Autodesk Fusion 360 part; units mm, degrees
(part 3 of 5)
sketch "Boceto1" plane through (0, 0, 0) normal (0, 1, 0) x (1, 0, 0)
  circle A0 centre (0, -615) radius 600 construction
  line L0 (0, 0) -> (-145, 0) construction
  circle A1 centre (-180, 0) radius 35 construction
  arc A2 (-148.5274, -15.3125) -> (-149.6891, 17.5) centre (-180, 0) ccw
  line L1 (-180, 0) -> (-153.1905, -22.5) construction
  line L2 (-180, 0) -> (-167.0096, 32.5) construction
  line L3 (-126.7013, 30.7139) -> (-107.5227, 7.8577)
  line L4 (-128.2, 32.5) -> (-139.7703, 32.5) construction
  line L5 (-138, 31.5) -> (-138, 5)
  line L6 (-138, 5) -> (-133.2, 5)
  line L7 (-133.2, 5) -> (-133.2, 31.25)
  line L8 (-141.0289, 32.5) -> (-139, 32.5)
  line L9 (-131.95, 32.5) -> (-130.5315, 32.5)
  line L10 (-145, 0) -> (-145, 32.5) construction
  line L11 (-35, -5) -> (-109.7758, -5)
  line L12 (-115.9041, -7.8577) -> (-125.7926, -19.6423)
  line L13 (-131.9209, -22.5) -> (-144.0313, -22.5)
  line L14 (-128.2, 19.2264) -> (-128.2, 7)
  line L15 (-126.2, 5) -> (-115.9408, 5)
  line L16 (-114.4087, 8.2856) -> (-124.6679, 20.512)
  arc A3 (-148.5274, -15.3125) -> (-144.0313, -22.5) centre (-144.0313, -17.5) ccw
  arc A4 (-141.0289, 32.5) -> (-149.6891, 17.5) centre (-141.0289, 22.5) ccw
  arc A5 (-128.2, 7) -> (-126.2, 5) centre (-126.2, 7) ccw
  arc A6 (-115.9408, 5) -> (-114.4087, 8.2856) centre (-115.9408, 7) ccw
  arc A7 (-124.6679, 20.512) -> (-128.2, 19.2264) centre (-126.2, 19.2264) ccw
  line L17 (-131.7, -16.1564) -> (-131.7, -1)
  line L18 (-129.934, -16.7992) -> (-117.2162, -1.6428)
  line L19 (-130.7, 0) -> (-117.9823, 0)
  arc A8 (-131.7, -16.1564) -> (-129.934, -16.7992) centre (-130.7, -16.1564) ccw
  arc A9 (-117.2162, -1.6428) -> (-117.9823, 0) centre (-117.9823, -1) ccw
  arc A10 (-130.7, 0) -> (-131.7, -1) centre (-130.7, -1) ccw
  line L20 (-138, 31.5) -> (-139, 32.5)
  line L21 (-133.2, 31.25) -> (-131.95, 32.5)
  arc A11 (-131.9209, -22.5) -> (-125.7926, -19.6423) centre (-131.9209, -14.5) ccw
  arc A12 (-109.7758, -5) -> (-115.9041, -7.8577) centre (-109.7758, -13) ccw
  arc A13 (-107.5227, 7.8577) -> (-101.3943, 5) centre (-101.3943, 13) ccw
  arc A14 (-126.7013, 30.7139) -> (-130.5315, 32.5) centre (-130.5315, 27.5) ccw
  line L22 (0, 105) -> (-30, 105)
  line L23 (-22, -14.9217) -> (-22, 0)
  line L24 (-22, 0) -> (-17.2, 0)
  line L25 (-17.2, 0) -> (-17.2, -14.7323)
  arc A15 (0, -15) -> (-16.6861, -15.2321) centre (0, -615) ccw
  arc A16 (-22.4813, -15.4213) -> (-26.8657, -15.6018) centre (0, -615) ccw
  line L26 (-30, -10) -> (-30, -12.6048)
  arc A17 (-30, -10) -> (-35, -5) centre (-35, -10) ccw
  arc A18 (-30, -12.6048) -> (-26.8657, -15.6018) centre (-27, -12.6048) ccw
  line L27 (0, 105) -> (0, -15)
  circle A19 centre (-143.9289, 24) radius 2.5
  circle A20 centre (-140.0313, -14.5) radius 4
  circle A21 centre (-138.0313, -4.5) radius 2.5
  line L28 (0, -1.75) -> (0, -22.5)
  arc A22 (149.6891, 17.5) -> (141.0289, 32.5) centre (141.0289, 22.5) ccw
  arc A23 (149.6891, 17.5) -> (148.5274, -15.3125) centre (180, 0) ccw
  circle A24 centre (143.9289, 24) radius 2.5
  line L29 (141.0289, 32.5) -> (139, 32.5)
  line L30 (138, 31.5) -> (139, 32.5)
  line L31 (138, 31.5) -> (138, 5)
  line L32 (133.2, 5) -> (133.2, 31.25)
  line L33 (138, 5) -> (133.2, 5)
  line L34 (133.2, 31.25) -> (131.95, 32.5)
  arc A25 (130.5315, 32.5) -> (126.7013, 30.7139) centre (130.5315, 27.5) ccw
  line L35 (131.95, 32.5) -> (130.5315, 32.5)
  arc A26 (128.2, 19.2264) -> (124.6679, 20.512) centre (126.2, 19.2264) ccw
  line L36 (128.2, 19.2264) -> (128.2, 7)
  line L37 (114.4087, 8.2856) -> (124.6679, 20.512)
  line L38 (126.7013, 30.7139) -> (107.5227, 7.8577)
  arc A27 (114.4087, 8.2856) -> (115.9408, 5) centre (115.9408, 7) ccw
  line L39 (126.2, 5) -> (115.9408, 5)
  arc A28 (126.2, 5) -> (128.2, 7) centre (126.2, 7) ccw
  circle A29 centre (138.0313, -4.5) radius 2.5
  arc A30 (131.7, -1) -> (130.7, 0) centre (130.7, -1) ccw
  line L40 (131.7, -16.1564) -> (131.7, -1)
  arc A31 (117.9823, 0) -> (117.2162, -1.6428) centre (117.9823, -1) ccw
  line L41 (130.7, 0) -> (117.9823, 0)
  line L42 (129.934, -16.7992) -> (117.2162, -1.6428)
  arc A32 (129.934, -16.7992) -> (131.7, -16.1564) centre (130.7, -16.1564) ccw
  circle A33 centre (140.0313, -14.5) radius 4
  arc A34 (144.0313, -22.5) -> (148.5274, -15.3125) centre (144.0313, -17.5) ccw
  line L43 (131.9209, -22.5) -> (144.0313, -22.5)
  arc A35 (125.7926, -19.6423) -> (131.9209, -22.5) centre (131.9209, -14.5) ccw
  line L44 (115.9041, -7.8577) -> (125.7926, -19.6423)
  arc A36 (115.9041, -7.8577) -> (109.7758, -5) centre (109.7758, -13) ccw
  line L45 (35, -5) -> (109.7758, -5)
  arc A37 (101.3943, 5) -> (107.5227, 7.8577) centre (101.3943, 13) ccw
  arc A38 (35, -5) -> (30, -10) centre (35, -10) ccw
  arc A39 (26.8657, -15.6018) -> (30, -12.6048) centre (27, -12.6048) ccw
  line L46 (30, -10) -> (30, -12.6048)
  arc A40 (26.8657, -15.6018) -> (22.4813, -15.4213) centre (0, -615) ccw
  line L47 (22, -14.9217) -> (22, 0)
  arc A41 (16.6861, -15.2321) -> (0, -15) centre (0, -615) ccw
  line L48 (17.2, 0) -> (17.2, -14.7323)
  line L49 (0, 0) -> (145, 0) construction
  line L50 (0, 105) -> (30, 105)
  line L51 (17.2, 0) -> (22, 0)
  arc A42 (-22.4813, -15.4213) -> (-22, -14.9217) centre (-22.5, -14.9217) ccw
  arc A43 (-17.2, -14.7323) -> (-16.6861, -15.2321) centre (-16.7, -14.7323) ccw
  arc A44 (16.6861, -15.2321) -> (17.2, -14.7323) centre (16.7, -14.7323) ccw
  arc A45 (22, -14.9217) -> (22.4813, -15.4213) centre (22.5, -14.9217) ccw
  line L52 (-22, -8) -> (-17.2, -8)
  line L53 (17.2, -8) -> (22, -8)
  line L54 (-52.8349, 8.75) -> (-34.6651, 40.2211)
  line L55 (-56.4434, 12.5) -> (-32.0096, 54.8205)
  line L56 (-101.3943, 5) -> (-69.4338, 5)
  line L57 (-50.6699, 5) -> (-32.5, 5)
  line L58 (-30, 105) -> (-30, 62.3205)
  line L59 (-30, 38.9711) -> (-30, 7.5)
  arc A46 (-69.4338, 5) -> (-56.4434, 12.5) centre (-69.4338, 20) ccw
  arc A47 (-32.0096, 54.8205) -> (-30, 62.3205) centre (-45, 62.3205) ccw
  arc A48 (-30, 38.9711) -> (-34.6651, 40.2211) centre (-32.5, 38.9711) ccw
  arc A49 (-32.5, 5) -> (-30, 7.5) centre (-32.5, 7.5) ccw
  arc A50 (-52.8349, 8.75) -> (-50.6699, 5) centre (-50.6699, 7.5) ccw
  line L60 (30, 105) -> (30, 62.3205)
  arc A51 (30, 62.3205) -> (32.0096, 54.8205) centre (45, 62.3205) ccw
  line L61 (56.4434, 12.5) -> (32.0096, 54.8205)
  arc A52 (34.6651, 40.2211) -> (30, 38.9711) centre (32.5, 38.9711) ccw
  line L62 (30, 38.9711) -> (30, 7.5)
  arc A53 (30, 7.5) -> (32.5, 5) centre (32.5, 7.5) ccw
  line L63 (50.6699, 5) -> (32.5, 5)
  arc A54 (50.6699, 5) -> (52.8349, 8.75) centre (50.6699, 7.5) ccw
  line L64 (52.8349, 8.75) -> (34.6651, 40.2211)
  arc A55 (56.4434, 12.5) -> (69.4338, 5) centre (69.4338, 20) ccw
  line L65 (101.3943, 5) -> (69.4338, 5)
  line L66 (50.6699, 5) -> (32.5, 5)
  point P0 (-167.0096, 32.5)
  point P1 (-138, 32.5)
  point P2 (-133.2, 32.5)
  point P3 (-128.1905, -22.5)
  point P4 (-30, 5)
  point P5 (-55, 5)
  dimension "d1" = 1200
  dimension "d13" = 70
  dimension "d21" = 50
  dimension "d23" = 5
  dimension "d25" = 4.8
  dimension "d26" = 7
  dimension "d27" = 5
  dimension "d28" = 5
  dimension "d29" = 25
  dimension "d30" = 50
  dimension "d31" = 55
  dimension "d32" = 32.5
  dimension "d33" = 5
  dimension "d34" = 5
  dimension "d35" = 10
  dimension "d36" = 2
  dimension "d37" = 32.5
  dimension "d39" = 5
  dimension "d40" = 1
  dimension "d44" = 1
  dimension "d45" = 1
  dimension "d46" = 1.25
  dimension "d47" = 1.25
  dimension "d48" = 8
  dimension "d49" = 5
  dimension "d50" = 5
  dimension "d52" = 30
  dimension "d53" = 600
  dimension "d54" = 4.8
  dimension "d55" = 8
  dimension "d57" = 5
  dimension "d58" = 3
  dimension "d59" = 120
  dimension "d72" = 1.5
  dimension "d73" = 5
  dimension "d74" = 2.9
  dimension "d75" = 1.5
  dimension "d76" = 8
  dimension "d78" = 4
  dimension "d79" = 3
  dimension "d80" = 5
  dimension "d81" = 10
  dimension "d82" = 2
  dimension "d83" = 615
  dimension "d84" = 0.5
  dimension "d85" = 7
  dimension "d86" = 7
  dimension "d87" = 60
  dimension "d88" = 25
  dimension "d89" = 5
  dimension "d90" = 15
  dimension "d91" = 2.5
  dimension "d166" = 180
  constraint coincident L0 A1.centre
  constraint coincident L0.end A1
  constraint coincident L49.start L0
  constraint coincident L0.start L49.start
  constraint coincident A1 P0
  constraint coincident A1.centre A2.centre
  constraint parallel L0 L8
  constraint horizontal L4
  constraint perpendicular L5 L8
  constraint perpendicular L5 L6
  constraint perpendicular L7 L9
  constraint collinear L8 L9
  constraint coincident L8 L10.end
  constraint tangent A2 L10
  constraint parallel L0 L11
  constraint horizontal L13
  constraint perpendicular L4 L14
  constraint perpendicular L14 L15
  constraint parallel L3 L16
  constraint coincident L6.end L15
  constraint coincident L4.start L14
  constraint coincident L1.end L13
  constraint coincident L1.end A2
  constraint tangent L13 A3
  constraint tangent A2 A3
  constraint coincident P0 L2.end
  constraint tangent L8 A4
  constraint tangent A2 A4
  constraint tangent L14 A5
  constraint tangent L15 A5
  constraint tangent L15 A6
  constraint tangent L16 A6
  constraint equal A5 A6
  constraint tangent L14 A7
  constraint tangent L16 A7
  constraint equal A5 A7
  constraint perpendicular L0 L17
  constraint parallel L12 L18
  constraint tangent L17 A8
  constraint tangent L18 A8
  constraint tangent L18 A9
  constraint tangent L19 A9
  constraint equal A8 A9
  constraint tangent L17 A10
  constraint tangent L19 A10
  constraint equal A8 A10
  constraint coincident L0 L19.start
  constraint horizontal L19
  constraint coincident P1 L5
  constraint coincident P1 L8
  constraint coincident P2 L7
  constraint coincident P2 L9
  constraint coincident P3 L12
  constraint coincident P3 L13
  constraint tangent L12 A11
  constraint tangent L13 A11
  constraint tangent L11 A12
  constraint tangent L12 A12
  constraint equal A11 A12
  constraint tangent L3 A13
  constraint tangent A13 L56
  constraint equal A11 A13
  constraint coincident L4.start L9
  constraint coincident L4.start L3
  constraint tangent L9 A14
  constraint tangent L3 A14
  constraint horizontal L22
  constraint vertical L58
  constraint coincident A0 A15.start
  constraint vertical L23
  constraint perpendicular L23 L24
  constraint vertical L25
  constraint concentric A15 A16
  constraint coincident L0.start L24
  constraint collinear L26 L59
  constraint tangent L11 A17
  constraint tangent L26 A17
  constraint tangent A16 A18
  constraint tangent L26 A18
  constraint coincident A15 L27.end
  constraint coincident L0.start L27
  constraint coincident A0.centre L28
  constraint vertical L27
  constraint symmetric L0.start L27 L49.start
  constraint symmetric L0.end L27 L49.end
  constraint symmetric A2 L27 A23
  constraint symmetric L5.end L27 L31.end
  constraint symmetric L6.end L27 L32.start
  constraint symmetric L13.end L27 A34.start
  constraint symmetric A2.start L27 A23.end
  constraint symmetric A3 L27 A34
  constraint symmetric L8.start L27 A22.end
  constraint symmetric A2.end L27 A22.start
  constraint symmetric A4 L27 A22
  constraint symmetric L14.end L27 L36.end
  constraint symmetric L15.start L27 L39.start
  constraint symmetric A5 L27 A28
  constraint symmetric L15.end L27 A27.end
  constraint symmetric L16.start L27 L37.start
  constraint symmetric A6 L27 A27
  constraint symmetric L14.start L27 A26.start
  constraint symmetric L16.end L27 A26.end
  constraint symmetric A7 L27 A26
  constraint symmetric L17.start L27 L40.start
  constraint symmetric L18.start L27 L42.start
  constraint symmetric A8 L27 A32
  constraint symmetric L18.end L27 A31.end
  constraint symmetric L19.end L27 A31.start
  constraint symmetric A9 L27 A31
  constraint symmetric L17.end L27 A30.start
  constraint symmetric L19.start L27 A30.end
  constraint symmetric A10 L27 A30
  constraint symmetric L5.start L27 L30.start
  constraint symmetric L8.end L27 L29.end
  constraint symmetric L7.end L27 L32.end
  constraint symmetric L9.start L27 L34.end
  constraint symmetric L12.end L27 A35.start
  constraint symmetric L13.start L27 L43.start
  constraint symmetric A11 L27 A35
  constraint symmetric L11.end L27 A36.end
  constraint symmetric L12.start L27 L44.start
  constraint symmetric A12 L27 A36
  constraint symmetric L3.end L27 L38.end
  constraint symmetric A13.end L27 A37.start
  constraint symmetric A13 L27 A37
  constraint symmetric L9.end L27 A25.start
  constraint symmetric L3.start L27 A25.end
  constraint symmetric A14 L27 A25
  constraint symmetric L22.end L27 L50.end
  constraint symmetric L23.end L27 L47.end
  constraint symmetric L24.end L27 L48.start
  constraint symmetric A15 L27 A41
  constraint symmetric A16 L27 A40
  constraint symmetric L11.start L27 L45.start
  constraint symmetric L26.start L27 A38.end
  constraint symmetric A17 L27 A38
  constraint symmetric L26.end L27 A39.end
  constraint symmetric A16.end L27 A39.start
  constraint symmetric A18 L27 A39
  constraint symmetric L22.start L27 L50.start
  constraint symmetric A15.start L27 A41.end
  constraint symmetric L27 A19 A24
  constraint symmetric L27 A20 A33
  constraint symmetric L27 A21 A29
  constraint tangent L23 A42
  constraint tangent A16 A42
  constraint tangent L25 A43
  constraint tangent A15 A43
  constraint equal A42 A43
  constraint tangent A41 A44
  constraint tangent L48 A44
  constraint equal A42 A44
  constraint tangent A40 A45
  constraint tangent L47 A45
  constraint equal A42 A45
  constraint vertical L48
  constraint vertical L47
  constraint equal A0 A16
  constraint coincident L23 L52.start
  constraint coincident L25 L52.end
  constraint perpendicular L25 L52
  constraint coincident L48 L53.start
  constraint coincident L47 L53.end
  constraint perpendicular L47 L53
  constraint coincident L23.end L24.start
  constraint parallel L54 L55
  constraint collinear L56 L57
  constraint collinear L58 L59
  constraint tangent L55 A46
  constraint tangent L56 A46
  constraint tangent L55 A47
  constraint tangent L58 A47
  constraint equal A46 A47
  constraint tangent L54 A48
  constraint tangent L59 A48
  constraint coincident P4 L57
  constraint tangent L57 A49
  constraint tangent L59 A49
  constraint equal A48 A49
  constraint coincident P5 L57
  constraint coincident P5 L54
  constraint tangent L57 A50
  constraint tangent L54 A50
  constraint equal A48 A50
  constraint coincident P4 L59
  constraint symmetric L27 L55.start L61.start
  constraint symmetric L27 L56.end A55.end
  constraint symmetric L27 A46 A55
  constraint symmetric L27 L55.end A51.end
  constraint symmetric L27 L58.end L60.end
  constraint symmetric L27 A47 A51
  constraint symmetric L27 L54.end A52.start
  constraint symmetric L27 L59.start A52.end
  constraint symmetric L27 A48 A52
  constraint symmetric L27 L57.end A53.end
  constraint symmetric L27 L59.end L62.end
  constraint symmetric L27 A49 A53
  constraint symmetric L27 L57.start L63.start
  constraint symmetric L27 L54.start A54.end
  constraint symmetric L27 A50 A54
  constraint collinear L65 L66
  measures "d1" diameter of A0
  measures "d13" diameter of A1
  measures "d21" angle of L3 L4
  measures "d23" distance of L0 L56
  measures "d25" distance of L5.end L6.end
  measures "d26" distance of L5 L10
  measures "d27" distance of L4.start L7
  measures "d28" distance of L0 L11
  measures "d29" distance of L1.end P3
  measures "d30" angle of L12 L13
  measures "d31" distance of L8 L13
  measures "d32" vertical distance of L0.end P0
  measures "d33" distance of L3 L16
  measures "d34" radius of A3
  measures "d35" radius of A4
  measures "d36" radius of A5
  measures "d37" distance of A1.centre L8
  measures "d39" distance of L12 L18
  measures "d40" radius of A8
  measures "d44" distance of P1 L5.start
  measures "d45" distance of P1 L8.end
  measures "d46" distance of P2 L7.end
  measures "d47" distance of P2 L9.start
  measures "d48" radius of A11
  measures "d49" radius of A14
  measures "d50" distance of L0 L6
  measures "d52" distance of L0.start L59
  measures "d53" radius of A15
  measures "d54" distance of L23.end L24.end
  measures "d55" distance of L23 L59
  measures "d57" radius of A17
  measures "d58" radius of A18
  measures "d59" distance of L22 A15.start
  measures "d72" distance of L7 L17
  measures "d73" diameter of A19
  measures "d74" horizontal distance of A4.centre A19.centre
  measures "d75" vertical distance of A4.centre A19.centre
  measures "d76" diameter of A20
  measures "d78" horizontal distance of A3.centre A20.centre
  measures "d79" vertical distance of A3.centre A20.centre
  measures "d80" diameter of A21
  measures "d81" vertical distance of A20.centre A21.centre
  measures "d82" horizontal distance of A20.centre A21.centre
  measures "d83" distance of L0.start A0.centre
  measures "d84" radius of A42
  measures "d85" distance of A15.start L52
  measures "d86" distance of A15.start L53
  measures "d87" angle of L54 L57
  measures "d88" distance of P4 P5
  measures "d89" distance of L54 L55
  measures "d90" radius of A46
  measures "d91" radius of A48
  measures "d166" horizontal distance of A1.centre L28.end
extrude "Extruir1" add sketch "Boceto1" along normal blind 4.8
sketch "Boceto2" plane through (0, 0, 0) normal (0, -1, 0) x (1, 0, 0)
  line L0 (-17.2, 14.7323) -> (-17.2, 8)
  line L1 (-22, 8) -> (-22, 14.9217)
  arc A0 (-16.6861, 15.2321) -> (16.6861, 15.2321) centre (0, 615) ccw
  arc A1 (-26.8657, 15.6018) -> (-30, 12.6048) centre (-27, 12.6048) ccw
  line L2 (-30, 12.6048) -> (-30, 10)
  arc A2 (-35, 5) -> (-30, 10) centre (-35, 10) ccw
  line L3 (-35, 5) -> (-109.7758, 5)
  arc A3 (-115.9041, 7.8577) -> (-109.7758, 5) centre (-109.7758, 13) ccw
  line L4 (-115.9041, 7.8577) -> (-125.7926, 19.6423)
  arc A4 (-125.7926, 19.6423) -> (-131.9209, 22.5) centre (-131.9209, 14.5) ccw
  line L5 (-131.9209, 22.5) -> (-144.0313, 22.5)
  arc A5 (-144.0313, 22.5) -> (-148.5274, 15.3125) centre (-144.0313, 17.5) ccw
  arc A6 (-149.6891, -17.5) -> (-148.5274, 15.3125) centre (-180, 0) ccw
  arc A7 (-149.6891, -17.5) -> (-141.0289, -32.5) centre (-141.0289, -22.5) ccw
  line L6 (-141.0289, -32.5) -> (-139, -32.5)
  line L7 (-139, -32.5) -> (-138, -31.5)
  line L8 (-138, -31.5) -> (-138, -5)
  line L9 (-138, -5) -> (-133.2, -5)
  line L10 (-133.2, -5) -> (-133.2, -31.25)
  line L11 (-133.2, -31.25) -> (-131.95, -32.5)
  line L12 (-131.95, -32.5) -> (-130.5315, -32.5)
  arc A8 (-130.5315, -32.5) -> (-126.7013, -30.7139) centre (-130.5315, -27.5) ccw
  line L13 (-126.7013, -30.7139) -> (-107.5227, -7.8577)
  arc A9 (-101.3943, -5) -> (-107.5227, -7.8577) centre (-101.3943, -13) ccw
  line L14 (-101.3943, -5) -> (-69.4338, -5)
  line L15 (-30, -62.3205) -> (-30, -105)
  line L16 (-30, -105) -> (30, -105)
  line L17 (0, 1.75) -> (0, 22.5)
  line L18 (8.6105, 15.0618) -> (4.2286, 3.0227)
  arc A10 (0, 9.0618) -> (4.2286, 3.0227) centre (0, 4.5618) ccw
  line L19 (8.6105, 15.0618) -> (-3.0966, 15.0618) construction
  arc A11 (0, 11.0618) -> (6.108, 2.3387) centre (0, 4.5618) ccw
  line L20 (6.108, 2.3387) -> (10.7514, 15.0963)
  arc A12 (0, 9.0618) -> (0, 11.0618) centre (0, 10.0618) ccw
  arc A13 (-22, 14.9217) -> (-22.4813, 15.4213) centre (-22.5, 14.9217) ccw
  arc A14 (-16.6861, 15.2321) -> (-17.2, 14.7323) centre (-16.7, 14.7323) ccw
  arc A15 (115.9408, -5) -> (114.4087, -8.2856) centre (115.9408, -7) ccw
  line L21 (115.9408, -5) -> (126.2, -5)
  arc A16 (128.2, -7) -> (126.2, -5) centre (126.2, -7) ccw
  line L22 (128.2, -7) -> (128.2, -19.2264)
  arc A17 (124.6679, -20.512) -> (128.2, -19.2264) centre (126.2, -19.2264) ccw
  line L23 (124.6679, -20.512) -> (114.4087, -8.2856)
  circle A18 centre (140.0313, 14.5) radius 4
  circle A19 centre (138.0313, 4.5) radius 2.5
  circle A20 centre (143.9289, -24) radius 2.5
  arc A21 (131.7, 16.1564) -> (129.934, 16.7992) centre (130.7, 16.1564) ccw
  line L24 (131.7, 16.1564) -> (131.7, 1)
  arc A22 (130.7, 0) -> (131.7, 1) centre (130.7, 1) ccw
  line L25 (130.7, 0) -> (117.9823, 0)
  arc A23 (117.2162, 1.6428) -> (117.9823, 0) centre (117.9823, 1) ccw
  line L26 (117.2162, 1.6428) -> (129.934, 16.7992)
  line L27 (17.2, 8) -> (17.2, 14.7323)
  arc A24 (17.2, 14.7323) -> (16.6861, 15.2321) centre (16.7, 14.7323) ccw
  arc A25 (-26.8657, 15.6018) -> (-22.4813, 15.4213) centre (0, 615) ccw
  line L28 (32.5, -5) -> (50.6699, -5)
  arc A26 (107.5227, -7.8577) -> (101.3943, -5) centre (101.3943, -13) ccw
  line L29 (107.5227, -7.8577) -> (126.7013, -30.7139)
  arc A27 (126.7013, -30.7139) -> (130.5315, -32.5) centre (130.5315, -27.5) ccw
  line L30 (130.5315, -32.5) -> (131.95, -32.5)
  line L31 (131.95, -32.5) -> (133.2, -31.25)
  line L32 (133.2, -31.25) -> (133.2, -5)
  line L33 (133.2, -5) -> (138, -5)
  line L34 (138, -5) -> (138, -31.5)
  line L35 (138, -31.5) -> (139, -32.5)
  line L36 (139, -32.5) -> (141.0289, -32.5)
  arc A28 (141.0289, -32.5) -> (149.6891, -17.5) centre (141.0289, -22.5) ccw
  arc A29 (148.5274, 15.3125) -> (149.6891, -17.5) centre (180, 0) ccw
  arc A30 (148.5274, 15.3125) -> (144.0313, 22.5) centre (144.0313, 17.5) ccw
  line L37 (144.0313, 22.5) -> (131.9209, 22.5)
  arc A31 (131.9209, 22.5) -> (125.7926, 19.6423) centre (131.9209, 14.5) ccw
  line L38 (125.7926, 19.6423) -> (115.9041, 7.8577)
  arc A32 (109.7758, 5) -> (115.9041, 7.8577) centre (109.7758, 13) ccw
  line L39 (109.7758, 5) -> (35, 5)
  arc A33 (30, 10) -> (35, 5) centre (35, 10) ccw
  line L40 (30, 10) -> (30, 12.6048)
  arc A34 (30, 12.6048) -> (26.8657, 15.6018) centre (27, 12.6048) ccw
  arc A35 (22.4813, 15.4213) -> (26.8657, 15.6018) centre (0, 615) ccw
  arc A36 (22.4813, 15.4213) -> (22, 14.9217) centre (22.5, 14.9217) ccw
  line L41 (22, 14.9217) -> (22, 8)
  line L42 (-17.2, 8) -> (-22, 8)
  line L43 (22, 8) -> (17.2, 8)
  arc A37 (52.8349, -8.75) -> (50.6699, -5) centre (50.6699, -7.5) ccw
  line L44 (52.8349, -8.75) -> (34.6651, -40.2211)
  arc A38 (30, -38.9711) -> (34.6651, -40.2211) centre (32.5, -38.9711) ccw
  line L45 (30, -38.9711) -> (30, -7.5)
  arc A39 (32.5, -5) -> (30, -7.5) centre (32.5, -7.5) ccw
  arc A40 (-56.4434, -12.5) -> (-69.4338, -5) centre (-69.4338, -20) ccw
  line L46 (-56.4434, -12.5) -> (-32.0096, -54.8205)
  arc A41 (-30, -62.3205) -> (-32.0096, -54.8205) centre (-45, -62.3205) ccw
  line L47 (30, -105) -> (30, -62.3205)
  arc A42 (32.0096, -54.8205) -> (30, -62.3205) centre (45, -62.3205) ccw
  line L48 (32.0096, -54.8205) -> (56.4434, -12.5)
  arc A43 (69.4338, -5) -> (56.4434, -12.5) centre (69.4338, -20) ccw
  line L49 (69.4338, -5) -> (101.3943, -5)
  arc A44 (-129.934, 16.7992) -> (-131.7, 16.1564) centre (-130.7, 16.1564) ccw
  line L50 (-129.934, 16.7992) -> (-117.2162, 1.6428)
  arc A45 (-117.9823, 0) -> (-117.2162, 1.6428) centre (-117.9823, 1) ccw
  line L51 (-117.9823, 0) -> (-130.7, 0)
  arc A46 (-131.7, 1) -> (-130.7, 0) centre (-130.7, 1) ccw
  line L52 (-131.7, 1) -> (-131.7, 16.1564)
  arc A47 (-34.6651, -40.2211) -> (-30, -38.9711) centre (-32.5, -38.9711) ccw
  line L53 (-34.6651, -40.2211) -> (-52.8349, -8.75)
  arc A48 (-50.6699, -5) -> (-52.8349, -8.75) centre (-50.6699, -7.5) ccw
  line L54 (-50.6699, -5) -> (-32.5, -5)
  arc A49 (-30, -7.5) -> (-32.5, -5) centre (-32.5, -7.5) ccw
  line L55 (-30, -7.5) -> (-30, -38.9711)
  arc A50 (-128.2, -19.2264) -> (-124.6679, -20.512) centre (-126.2, -19.2264) ccw
  line L56 (-128.2, -19.2264) -> (-128.2, -7)
  arc A51 (-126.2, -5) -> (-128.2, -7) centre (-126.2, -7) ccw
  line L57 (-126.2, -5) -> (-115.9408, -5)
  arc A52 (-114.4087, -8.2856) -> (-115.9408, -5) centre (-115.9408, -7) ccw
  line L58 (-114.4087, -8.2856) -> (-124.6679, -20.512)
  circle A53 centre (-138.0313, 4.5) radius 2.5
  circle A54 centre (-143.9289, -24) radius 2.5
  circle A55 centre (-140.0313, 14.5) radius 4
  dimension "d7" = 350
  dimension "d8" = 175
  dimension "d65" = 2
  dimension "d66" = 70
  dimension "d67" = 2
  dimension "d69" = 4.5
  dimension "d71" = 5
  constraint coincident A12.centre L17
  constraint tangent L18 A10
  constraint tangent A10 A12
  constraint horizontal L19
  constraint tangent A11 L20
  constraint parallel L18 L20
  constraint coincident L17 A10.centre
  constraint coincident A0 L18.start
  constraint coincident A0 L20.end
  measures "d65" diameter of A12
  measures "d66" angle of L18 L19
  measures "d69" radius of A10
  measures "d71" distance of A12.centre L19
extrude "Extruir2" cut sketch "Boceto2" against normal through all contours A0 L17 L18 A10 A11 L20 | L17 A12
sketch "Boceto4" plane through (0, 0, 0) normal (0, -1, 0) x (1, 0, 0)
  line L0 (10.7514, 15.0963) -> (6.108, 2.3387)
  arc A0 (0, 11.0618) -> (6.108, 2.3387) centre (0, 4.5618) ccw
  arc A1 (0, 9.0618) -> (0, 11.0618) centre (0, 10.0618) ccw
  arc A2 (0, 9.0618) -> (4.2286, 3.0227) centre (0, 4.5618) ccw
  line L1 (4.2286, 3.0227) -> (8.6105, 15.0618)
  arc A3 (-16.6861, 15.2321) -> (8.6105, 15.0618) centre (0, 615) ccw
  arc A4 (-16.6861, 15.2321) -> (-17.2, 14.7323) centre (-16.7, 14.7323) ccw
  line L2 (-17.2, 14.7323) -> (-17.2, 8)
  line L3 (-17.2, 8) -> (-22, 8)
  line L4 (-22, 8) -> (-22, 14.9217)
  arc A5 (-22, 14.9217) -> (-22.4813, 15.4213) centre (-22.5, 14.9217) ccw
  arc A6 (-26.8657, 15.6018) -> (-22.4813, 15.4213) centre (0, 615) ccw
  arc A7 (-26.8657, 15.6018) -> (-30, 12.6048) centre (-27, 12.6048) ccw
  line L5 (-30, 12.6048) -> (-30, 10)
  arc A8 (-35, 5) -> (-30, 10) centre (-35, 10) ccw
  line L6 (-35, 5) -> (-109.7758, 5)
  arc A9 (-115.9041, 7.8577) -> (-109.7758, 5) centre (-109.7758, 13) ccw
  line L7 (-115.9041, 7.8577) -> (-125.7926, 19.6423)
  arc A10 (-125.7926, 19.6423) -> (-131.9209, 22.5) centre (-131.9209, 14.5) ccw
  line L8 (-131.9209, 22.5) -> (-144.0313, 22.5)
  arc A11 (-144.0313, 22.5) -> (-148.5274, 15.3125) centre (-144.0313, 17.5) ccw
  arc A12 (-149.6891, -17.5) -> (-148.5274, 15.3125) centre (-180, 0) ccw
  arc A13 (-149.6891, -17.5) -> (-141.0289, -32.5) centre (-141.0289, -22.5) ccw
  line L9 (-141.0289, -32.5) -> (-139, -32.5)
  line L10 (-139, -32.5) -> (-138, -31.5)
  line L11 (-138, -31.5) -> (-138, -5)
  line L12 (-138, -5) -> (-133.2, -5)
  line L13 (-133.2, -5) -> (-133.2, -31.25)
  line L14 (-133.2, -31.25) -> (-131.95, -32.5)
  line L15 (-131.95, -32.5) -> (-130.5315, -32.5)
  arc A14 (-130.5315, -32.5) -> (-126.7013, -30.7139) centre (-130.5315, -27.5) ccw
  line L16 (-126.7013, -30.7139) -> (-107.5227, -7.8577)
  arc A15 (-101.3943, -5) -> (-107.5227, -7.8577) centre (-101.3943, -13) ccw
  line L17 (-101.3943, -5) -> (-69.4338, -5)
  arc A16 (-56.4434, -12.5) -> (-69.4338, -5) centre (-69.4338, -20) ccw
  line L18 (-56.4434, -12.5) -> (-32.0096, -54.8205)
  arc A17 (-30, -62.3205) -> (-32.0096, -54.8205) centre (-45, -62.3205) ccw
  line L19 (-30, -62.3205) -> (-30, -105)
  line L20 (-30, -105) -> (30, -105)
  line L21 (30, -105) -> (30, -62.3205)
  arc A18 (32.0096, -54.8205) -> (30, -62.3205) centre (45, -62.3205) ccw
  line L22 (32.0096, -54.8205) -> (56.4434, -12.5)
  arc A19 (69.4338, -5) -> (56.4434, -12.5) centre (69.4338, -20) ccw
  line L23 (69.4338, -5) -> (101.3943, -5)
  arc A20 (107.5227, -7.8577) -> (101.3943, -5) centre (101.3943, -13) ccw
  line L24 (107.5227, -7.8577) -> (126.7013, -30.7139)
  arc A21 (126.7013, -30.7139) -> (130.5315, -32.5) centre (130.5315, -27.5) ccw
  line L25 (130.5315, -32.5) -> (131.95, -32.5)
  line L26 (131.95, -32.5) -> (133.2, -31.25)
  line L27 (133.2, -31.25) -> (133.2, -5)
  line L28 (133.2, -5) -> (138, -5)
  line L29 (138, -5) -> (138, -31.5)
  line L30 (138, -31.5) -> (139, -32.5)
  line L31 (139, -32.5) -> (141.0289, -32.5)
  arc A22 (141.0289, -32.5) -> (149.6891, -17.5) centre (141.0289, -22.5) ccw
  arc A23 (148.5274, 15.3125) -> (149.6891, -17.5) centre (180, 0) ccw
  arc A24 (148.5274, 15.3125) -> (144.0313, 22.5) centre (144.0313, 17.5) ccw
  line L32 (144.0313, 22.5) -> (131.9209, 22.5)
  arc A25 (131.9209, 22.5) -> (125.7926, 19.6423) centre (131.9209, 14.5) ccw
  line L33 (125.7926, 19.6423) -> (115.9041, 7.8577)
  arc A26 (109.7758, 5) -> (115.9041, 7.8577) centre (109.7758, 13) ccw
  line L34 (109.7758, 5) -> (35, 5)
  arc A27 (30, 10) -> (35, 5) centre (35, 10) ccw
  line L35 (30, 10) -> (30, 12.6048)
  arc A28 (30, 12.6048) -> (26.8657, 15.6018) centre (27, 12.6048) ccw
  arc A29 (22.4813, 15.4213) -> (26.8657, 15.6018) centre (0, 615) ccw
  arc A30 (22.4813, 15.4213) -> (22, 14.9217) centre (22.5, 14.9217) ccw
  line L36 (22, 14.9217) -> (22, 8)
  line L37 (22, 8) -> (17.2, 8)
  line L38 (17.2, 8) -> (17.2, 14.7323)
  arc A31 (17.2, 14.7323) -> (16.6861, 15.2321) centre (16.7, 14.7323) ccw
  arc A32 (10.7514, 15.0963) -> (16.6861, 15.2321) centre (0, 615) ccw
  circle A33 centre (-140.0313, 14.5) radius 4
  circle A34 centre (138.0313, 4.5) radius 2.5
  circle A35 centre (-143.9289, -24) radius 2.5
  arc A36 (131.7, 16.1564) -> (129.934, 16.7992) centre (130.7, 16.1564) ccw
  line L39 (131.7, 16.1564) -> (131.7, 1)
  arc A37 (130.7, 0) -> (131.7, 1) centre (130.7, 1) ccw
  line L40 (130.7, 0) -> (117.9823, 0)
  arc A38 (117.2162, 1.6428) -> (117.9823, 0) centre (117.9823, 1) ccw
  line L41 (117.2162, 1.6428) -> (129.934, 16.7992)
  arc A39 (-129.934, 16.7992) -> (-131.7, 16.1564) centre (-130.7, 16.1564) ccw
  line L42 (-129.934, 16.7992) -> (-117.2162, 1.6428)
  arc A40 (-117.9823, 0) -> (-117.2162, 1.6428) centre (-117.9823, 1) ccw
  line L43 (-117.9823, 0) -> (-130.7, 0)
  arc A41 (-131.7, 1) -> (-130.7, 0) centre (-130.7, 1) ccw
  line L44 (-131.7, 1) -> (-131.7, 16.1564)
  circle A42 centre (143.9289, -24) radius 2.5
  arc A43 (115.9408, -5) -> (114.4087, -8.2856) centre (115.9408, -7) ccw
  line L45 (115.9408, -5) -> (126.2, -5)
  arc A44 (128.2, -7) -> (126.2, -5) centre (126.2, -7) ccw
  line L46 (128.2, -7) -> (128.2, -19.2264)
  arc A45 (124.6679, -20.512) -> (128.2, -19.2264) centre (126.2, -19.2264) ccw
  line L47 (124.6679, -20.512) -> (114.4087, -8.2856)
  line L48 (52.8349, -8.75) -> (34.6651, -40.2211)
  arc A46 (30, -38.9711) -> (34.6651, -40.2211) centre (32.5, -38.9711) ccw
  line L49 (30, -38.9711) -> (30, -7.5)
  arc A47 (32.5, -5) -> (30, -7.5) centre (32.5, -7.5) ccw
  line L50 (32.5, -5) -> (50.6699, -5)
  arc A48 (52.8349, -8.75) -> (50.6699, -5) centre (50.6699, -7.5) ccw
  arc A49 (-128.2, -19.2264) -> (-124.6679, -20.512) centre (-126.2, -19.2264) ccw
  line L51 (-128.2, -19.2264) -> (-128.2, -7)
  arc A50 (-126.2, -5) -> (-128.2, -7) centre (-126.2, -7) ccw
  line L52 (-126.2, -5) -> (-115.9408, -5)
  arc A51 (-114.4087, -8.2856) -> (-115.9408, -5) centre (-115.9408, -7) ccw
  line L53 (-114.4087, -8.2856) -> (-124.6679, -20.512)
  arc A52 (-34.6651, -40.2211) -> (-30, -38.9711) centre (-32.5, -38.9711) ccw
  line L54 (-34.6651, -40.2211) -> (-52.8349, -8.75)
  arc A53 (-50.6699, -5) -> (-52.8349, -8.75) centre (-50.6699, -7.5) ccw
  line L55 (-50.6699, -5) -> (-32.5, -5)
  arc A54 (-30, -7.5) -> (-32.5, -5) centre (-32.5, -7.5) ccw
  line L56 (-30, -7.5) -> (-30, -38.9711)
  circle A55 centre (140.0313, 14.5) radius 4
  circle A56 centre (-138.0313, 4.5) radius 2.5
  line L57 (-30, -63.3205) -> (-16, -63.3205)
  line L58 (-16, -63.3205) -> (-16, -68.1205)
  line L59 (-16, -68.1205) -> (-30, -68.1205)
  line L60 (0, -105) -> (0, 15)
  line L61 (16, -68.1205) -> (30, -68.1205)
  line L62 (30, -63.3205) -> (16, -63.3205)
  line L63 (16, -63.3205) -> (16, -68.1205)
  line L64 (-21, -5) -> (0, -5)
  line L65 (-21, -5) -> (-21, -30)
  line L66 (-21, -30) -> (0, -30)
  line L67 (-4, -36) -> (-4, -51.5233)
  line L68 (-4, -51.5233) -> (-22.5, -36)
  line L69 (-22.5, -36) -> (-4, -36)
  line L70 (-22.5, -43.8324) -> (-6.4256, -57.3205)
  line L71 (-22.5, -57.3205) -> (-22.5, -43.8324)
  line L72 (-22.5, -57.3205) -> (-6.4256, -57.3205)
  line L73 (22.5, -57.3205) -> (6.4256, -57.3205)
  line L74 (22.5, -43.8324) -> (6.4256, -57.3205)
  line L75 (22.5, -57.3205) -> (22.5, -43.8324)
  line L76 (4, -51.5233) -> (22.5, -36)
  line L77 (4, -36) -> (4, -51.5233)
  line L78 (22.5, -36) -> (4, -36)
  line L79 (21, -30) -> (0, -30)
  line L80 (21, -5) -> (21, -30)
  line L81 (21, -5) -> (0, -5)
  dimension "d92" = 4.8
  dimension "d93" = 14
  dimension "d94" = 1
  dimension "d98" = 9
  dimension "d102" = 6
  dimension "d103" = 6
  dimension "d104" = 8
  dimension "d105" = 40
  dimension "d110" = 25
  dimension "d111" = 7.5
  dimension "d112" = 6
  constraint coincident L19 L57.start
  constraint perpendicular L19 L57
  constraint perpendicular L57 L58
  constraint coincident L19 L59.end
  constraint perpendicular L19 L59
  constraint midpoint L20 L60.start
  constraint coincident A3 L60.end
  constraint perpendicular L20 L60
  constraint symmetric L57.start L60 L62.start
  constraint symmetric L57.end L60 L62.end
  constraint symmetric L58.end L60 L61.start
  constraint symmetric L59.end L60 L61.end
  constraint coincident L60 L64.end
  constraint perpendicular L60 L64
  constraint coincident L55 L64.start
  constraint parallel L60 L65
  constraint perpendicular L65 L66
  constraint perpendicular L66 L67
  constraint perpendicular L67 L69
  constraint vertical L71
  constraint parallel L68 L70
  constraint coincident L68.end L71
  constraint coincident L60 L66.end
  constraint horizontal L72
  constraint symmetric L60 L64.end L81.end
  constraint symmetric L60 L64.start L80.start
  constraint symmetric L60 L65.end L79.start
  constraint symmetric L60 L66.end L79.end
  constraint symmetric L60 L67.start L77.start
  constraint symmetric L60 L67.end L76.start
  constraint symmetric L60 L68.end L76.end
  constraint symmetric L60 L70.start L74.start
  constraint symmetric L60 L71.start L73.start
  constraint symmetric L60 L70.end L73.end
  measures "d92" distance of L57.end L58.end
  measures "d93" distance of L58.end L59.end
  measures "d94" distance of A17.start L57.start
  measures "d98" distance of L56 L65
  measures "d102" distance of L68 L70
  measures "d103" distance of L66 L69
  measures "d105" angle of L68 L69
  measures "d110" distance of L64.start L65.end
  measures "d111" distance of L56 L68.end
  measures "d112" distance of L57 L72
extrude "Extruir3" cut sketch "Boceto4" against normal blind 10 contours L60 L79 L80 L81 | L60 L64 L65 L66 | L19 L57 L58 L59 | L21 L61 L62 L63 | L67 L68 L69 | L70 L71 L72 | L73 L74 L75 | L76 L77 L78
chamfer "Chaflán1" distance 4 angle 45 4 edges at (-21, 2.4, -30) (-21, 2.4, -5) (21, 2.4, -5) (21, 2.4, -30)
fillet "Empalme3" radius 2 20 edges at (-17, 2.4, -30) (-21, 2.4, -26) (-21, 2.4, -9) (-17, 2.4, -5) (17, 2.4, -5) (21, 2.4, -9) (21, 2.4, -26) (17, 2.4, -30) (-22.5, 2.4, -36) (-4, 2.4, -36) (-4, 2.4, -51.5233) (-6.4256, 2.4, -57.3205) (-22.5, 2.4, -57.3205) (-22.5, 2.4, -43.8324) (22.5, 2.4, -57.3205) (6.4256, 2.4, -57.3205) (22.5, 2.4, -43.8324) (4, 2.4, -51.5233) (4, 2.4, -36) (22.5, 2.4, -36)